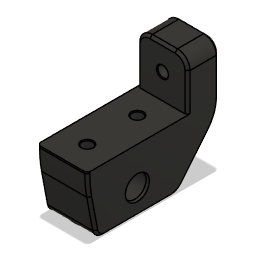
wheel stand hinge point v8 (Autodesk Fusion 360 design; units mm, degrees)
Autodesk Fusion 360 part; units mm, degrees
sketch "Sketch7" plane through (0, 0, 0) normal (1, 0, 0) x (0, 0, -1)
  line L0 (-40, 0) -> (40, 0)
  line L1 (40, 0) -> (40, 40)
  line L2 (40, 40) -> (65, 40)
  line L3 (65, 40) -> (65, -10)
  line L4 (-40, 0) -> (-40, -10)
  line L5 (0, 0) -> (0, -30) construction
  circle A0 centre (0, -30) radius 9.025
  line L6 (-40, -10) -> (-32.5, -50)
  line L7 (-32.5, -50) -> (32.5, -50)
  line L8 (32.5, -50) -> (65, -10)
  dimension "d98" = 80
  dimension "d99" = 40
  dimension "d100" = 25
  dimension "d101" = 50
  dimension "d102" = 10
  dimension "d103" = 30
  dimension "d104" = 18.05
  dimension "d105" = 7.5
  dimension "d106" = 7.5
  dimension "d107" = 50
  constraint horizontal L0
  constraint midpoint L5.start L0
  constraint perpendicular L0 L1
  constraint perpendicular L1 L2
  constraint perpendicular L2 L3
  constraint perpendicular L0 L4
  constraint coincident L5.start origin
  constraint perpendicular L0 L5
  constraint coincident L5.end A0.centre
  constraint horizontal L7
  measures "d98" distance of L0.start L0.end
  measures "d99" distance of L0.end L1.end
  measures "d100" distance of L1.end L2.end
  measures "d101" distance of L2.end L3.end
  measures "d102" distance of L0.start L4.end
  measures "d103" distance of L5.start L5.end
  measures "d104" diameter of A0
  measures "d105" horizontal distance of L0.start L6.end
  measures "d106" horizontal distance of L0.end L7.end
  measures "d107" distance of L0 L7
extrude "Extrude12" add sketch "Sketch7" along normal blind 40 makes body 1
sketch "Sketch8" plane through (0, 0, 0) normal (0, 1, 0) x (-1, 0, 0)
  line L0 (0, -40) -> (0, 40)
  line L1 (0, 40) -> (-40, 40)
  line L2 (-40, 40) -> (-40, -40)
  line L3 (-40, -40) -> (0, -40)
  line L4 (-40, 20) -> (0, 20) construction
  line L5 (0, -20) -> (-40, -20) construction
  circle A0 centre (-20, 20) radius 10.5
  circle A1 centre (-20, 20) radius 4.25
  circle A2 centre (-20, -20) radius 10.5
  circle A3 centre (-20, -20) radius 4.25
  dimension "d110" = 20
  dimension "d111" = 20
  dimension "d112" = 21
  dimension "d113" = 8.5
  constraint coincident L2 L4.start
  constraint coincident L0 L4.end
  constraint perpendicular L0 L4
  constraint coincident L0 L5.start
  constraint coincident L2 L5.end
  constraint perpendicular L2 L5
  constraint midpoint L4 A0.centre
  constraint concentric A0 A1
  constraint midpoint L5 A2.centre
  constraint concentric A2 A3
  constraint equal A1 A3
  constraint equal A0 A2
  measures "d110" distance of L3 L5
  measures "d111" distance of L1 L4
  measures "d112" diameter of A0
  measures "d113" diameter of A1
extrude "Extrude13" cut sketch "Sketch8" against normal blind 65 contours A0 | A1 | A2 | A3 bodies 1
extrude "Extrude14" add sketch "Sketch8" against normal blind 48 contours A0 | A2 bodies 1
sketch "Sketch9" plane through (0, 0, -40) normal (0, 0, 1) x (1, 0, 0)
  line L0 (0, 40) -> (0, 0)
  line L1 (0, 0) -> (40, 0)
  line L2 (40, 0) -> (40, 40)
  line L3 (40, 40) -> (0, 40)
  line L4 (0, 40) -> (40, 0) construction
  circle A0 centre (20, 20) radius 10.5
  circle A1 centre (20, 20) radius 4.25
  dimension "d118" = 21
  dimension "d119" = 8.5
  constraint coincident L0.start L3.end
  constraint coincident L1.end L2.start
  constraint midpoint L4 A0.centre
  constraint concentric A0 A1
  measures "d118" diameter of A0
  measures "d119" diameter of A1
extrude "Extrude15" cut sketch "Sketch9" against normal blind 25 contours A0 | A1 bodies 1
extrude "Extrude16" add sketch "Sketch9" against normal blind 20 contours A0 bodies 1
fillet "Fillet6" radius 7.5 1 edges at (20, -50, 32.5) on bodies 1
fillet "Fillet6" radius 92.5 1 edges at (20, -10, 40) on bodies 1
fillet "Fillet6" radius 12.5 1 edges at (20, -50, -32.5) on bodies 1
fillet "Fillet6" radius 32.5 1 edges at (20, -10, -65) on bodies 1
fillet "Fillet6" radius 10 2 edges at (40, 40, -52.5) (0, 40, -52.5) on bodies 1
chamfer "Chamfer2" distance 2 distance2 2 26 edges at (40, 15.7694, -65) (37.0711, 37.0711, -65) (20, 40, -65) (2.9289, 37.0711, -65) (0, 15.7694, -65) (0, -9.335, -63.127) (0, -32.1689, -46.9877) (0, -48.7867, -31.9225) (0, -50, -0.1374) (0, -48.2713, 31.0653) (0, -31.1659, 36.0314) (0, -9.9631, 39.6031) (0, -0.7015, 40) (40, -0.7015, 40) (40, -9.9631, 39.6031) (40, -31.1659, 36.0314) (40, -48.2713, 31.0653) (40, -50, -0.1374) (40, -48.7867, -31.9225) (40, -32.1689, -46.9877) (40, -9.335, -63.127) (37.0711, 37.0711, -40) (40, 15, -40) (0, 15, -40) (2.9289, 37.0711, -40) (20, 40, -40) measured on face at (40, -24.2407, -28.2919) measured on face at (30.9506, 39.9547, -56.6667) measured on face at (36.7942, 16.658, -65) measured on face at (0.0113, 30.4758, -48.3333) measured on face at (0, -24.2407, -28.2919) measured on face at (26.6667, -8.6357, -63.3663) measured on face at (26.6667, -36.5734, -43.4091) measured on face at (13.3333, -45.8515, -35.8511) measured on face at (36.4044, -50, -5.0795) measured on face at (20.063, -47.9696, 31.4072) measured on face at (13.3333, -26.9272, 36.8261) measured on face at (26.6667, -10.911, 39.51) measured on face at (26.6667, -0.9354, 40) measured on face at (40, -24.2407, -28.2919) measured on face at (26.6667, -10.911, 39.51) measured on face at (40, -24.2407, -28.2919) measured on face at (20.063, -47.9696, 31.4072) measured on face at (40, -24.2407, -28.2919) measured on face at (13.3333, -45.8515, -35.8511) measured on face at (40, -24.2407, -28.2919) measured on face at (26.6667, -8.6357, -63.3663) measured on face at (30.9506, 39.9547, -56.6667) measured on face at (40, -24.2407, -28.2919) measured on face at (0, -24.2407, -28.2919) measured on face at (0.0113, 30.4758, -48.3333) measured on face at (16.6667, 40, -48.3333) on bodies 1
chamfer "Chamfer2" distance 0.6 distance2 0.6 3 faces at (24.2447, 19.7882, -53.3333) (15.7553, -32, -20.2118) (15.7553, -32, 19.7882) on bodies 1
chamfer "Chamfer2" distance 0.6 distance2 2 1 edges at (40, -26.7364, 8.4143) measured on face at (40, -24.2407, -28.2919) on bodies 1
chamfer "Chamfer2" distance 2 distance2 0.6 1 edges at (0, -26.7364, 8.4143) measured on face at (26.6667, -30.4499, -9.0138) on bodies 1
copy_body "Body->Comp2" bodies 1 removing the originals makes body 2 in component "wheel stand hinge point"
component "wheel stand hinge point" placed x (1, 0, 0) y (0, 1, 0) z (0, 0, 1) at (0, 0, 0)
named bodies: "wheel stand hinge point"
